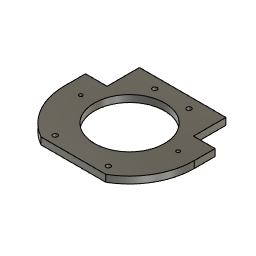
Lid (Autodesk Fusion 360 design; units mm, degrees)
Autodesk Fusion 360 part; units mm, degrees
sketch "Sketch1" plane through (0, 0, 0) normal (0, 0, 1) x (1, 0, 0)
  line L0 (0, 49.25) -> (40, 49.25)
  line L1 (40, 49.25) -> (40, 19.25)
  line L2 (40, 19.25) -> (60, 19.25)
  line L3 (60, 19.25) -> (60, 0)
  line L4 (0, -52) -> (30, -52)
  arc A0 (30, -52) -> (60, 0) centre (-0.0667, 0) ccw
  circle A1 centre (15.875, 39.25) radius 2.1
  circle A2 centre (45, 0) radius 1.6
  circle A3 centre (24.6, -44.1599) radius 2.1
  circle A4 centre (-45, 0) radius 1.6
  line L5 (-60, 14.25) -> (-60, 0)
  arc A5 (-60, 0) -> (-30, -52) centre (0.0667, 0) ccw
  line L6 (0, -52) -> (-30, -52)
  line L7 (0, 49.25) -> (-40, 49.25)
  circle A6 centre (0.0667, 0) radius 32.5
  line L8 (-40, 49.25) -> (-40, 19.25)
  line L9 (-40, 19.25) -> (-60, 19.25)
  line L10 (-60, 19.25) -> (-60, 14.25)
  circle A7 centre (-24.6, -44.1599) radius 2.1
  circle A8 centre (-15.875, 39.25) radius 2.1
  dimension "d1" = 49.25
  dimension "d2" = 40
  dimension "d3" = 30
  dimension "d4" = 20
  dimension "d5" = 52
  dimension "d6" = 30
  dimension "d12" = 4.2
  dimension "d13" = 45
  dimension "d14" = 3.2
  dimension "d17" = 4.2
  dimension "d20" = 65
  dimension "d23" = 30
  dimension "d24" = 4.2
  dimension "d25" = 4.2
  constraint perpendicular L0 L1
  constraint perpendicular L1 L2
  constraint perpendicular L2 L3
  constraint tangent L3 A0
  constraint concentric A5 A6
  constraint perpendicular L7 L8
  constraint perpendicular L8 L9
  constraint perpendicular L9 L10
  measures "d1" distance of origin L0.start
  measures "d2" distance of L0.start L0.end
  measures "d3" distance of L0.end L1.end
  measures "d4" distance of L1.end L2.end
  measures "d5" distance of origin L4.start
  measures "d6" distance of L4.start L4.end
  measures "d12" diameter of A1
  measures "d13" distance of origin A2.centre
  measures "d14" diameter of A2
  measures "d17" diameter of A3
  measures "d20" diameter of A6
  measures "d23" distance of L7.end L8.end
  measures "d24" diameter of A7
  measures "d25" diameter of A8
extrude "Extrude4" add sketch "Sketch1" along normal blind 6.35
